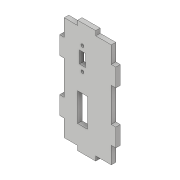
# Autodesk Inventor part: costat4
Saved by Autodesk Inventor 2019 (Build 230136000, 136)
## iProperties
Created: 2018-09-21
Part Number: costat4
Material: Genérico
Document SubType Name: Modeling
Designer: lmacia
Density: 1 g/cm^3
Appearance: Valor por defecto
Author: lmacia
Autodesk Inventor part; units mm, degrees
ref_plane "YZ Plane" through (0, 0, 0) normal (1, 0, 0) x (0, 1, 0)
ref_plane "XZ Plane" through (0, 0, 0) normal (0, 1, 0) x (-1, 0, 0)
ref_plane "XY Plane" through (0, 0, 0) normal (0, 0, 1) x (1, 0, 0)
sketch "Boceto1" plane through (0, 0, 0) normal (0, 0, 1) x (-1, 0, 0)
  line L0 (-15.8834, -11.4122) -> (-18.9334, -11.4122)
  line L1 (-18.9334, -11.4122) -> (-18.9334, -23.6123)
  line L2 (-18.9334, -23.6123) -> (-15.8834, -23.6123)
  line L3 (-15.8834, -23.6123) -> (-15.8834, -35.0245)
  line L4 (-15.8834, -35.0245) -> (-5.3608, -35.0245)
  line L5 (-5.3608, -35.0245) -> (-5.3608, -38.0745)
  line L6 (-5.3608, -38.0745) -> (6.8394, -38.0745)
  line L7 (6.8394, -38.0745) -> (6.8394, -35.0245)
  line L8 (6.8394, -35.0245) -> (15.8369, -35.0245)
  line L9 (15.8369, -35.0245) -> (15.8369, -23.6132)
  line L10 (15.8369, -23.6132) -> (18.887, -23.6123)
  line L11 (18.887, -23.6123) -> (18.887, -11.4122)
  line L12 (18.887, -11.4122) -> (15.8369, -11.4122)
  line L13 (15.8369, -11.4122) -> (15.8369, 11.4122)
  line L14 (15.8369, 11.4122) -> (18.887, 11.4122)
  line L15 (18.887, 11.4122) -> (18.887, 23.6123)
  line L16 (18.887, 23.6123) -> (15.8369, 23.6123)
  line L17 (15.8369, 23.6123) -> (15.8369, 28.9245)
  line L18 (15.8369, 28.9245) -> (15.8369, 35.0245)
  line L19 (15.8369, 35.0245) -> (6.8394, 35.0245)
  line L20 (6.8394, 35.0245) -> (6.8394, 38.0746)
  line L21 (6.8394, 38.0746) -> (-5.3608, 38.0746)
  line L22 (-5.3608, 38.0746) -> (-5.3608, 35.0245)
  line L23 (-5.3608, 35.0245) -> (-14.3584, 35.0245)
  line L24 (-14.3584, 35.0245) -> (-14.8667, 35.0245)
  line L25 (-14.8667, 35.0245) -> (-15.8834, 35.0245)
  line L26 (-15.8834, 35.0245) -> (-15.8834, 23.6123)
  line L27 (-15.8834, 23.6123) -> (-18.9334, 23.6123)
  line L28 (-18.9334, 23.6123) -> (-18.9334, 11.4122)
  line L29 (-18.9334, 11.4122) -> (-15.8834, 11.4122)
  line L30 (-15.8834, 11.4122) -> (-15.8834, -11.4122)
  line L31 (5.5685, -21.2994) -> (1.5018, -21.2994)
  line L32 (1.5018, -21.2994) -> (1.5018, -13.166)
  line L33 (1.5018, -13.166) -> (5.5685, -13.166)
  line L34 (5.5685, -13.166) -> (5.5685, -21.2994)
  line L35 (0.231, 3.1009) -> (0.231, 22.2144)
  line L36 (0.231, 22.2144) -> (6.8394, 22.2144)
  line L37 (6.8394, 22.2144) -> (6.8394, 3.1009)
  line L38 (6.8394, 3.1009) -> (0.231, 3.1009)
  circle A0 centre (3.5352, -9.6076) radius 1.0167
  circle A1 centre (3.5352, -24.8577) radius 1.0167
  point P0 (0, 0)
  dimension "d2" = 37.82
  dimension "d3" = 76.149
  constraints: 78 end point, 2 centre point
  measures "d3" distance between parallel lines of L21 L6
extrude "Extrusión1" add sketch "Boceto1" along normal blind 3
